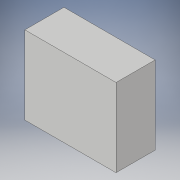
# Autodesk Inventor part: Tete
Saved by Autodesk Inventor 2019 (Build 230136000, 136)
## iProperties
Created: 2020-05-14
Part Number: Tete
Material: Générique
Document SubType Name: Modeling
Designer: qrrim
Density: 1 g/cm^3
Appearance: Par défaut
Author: qrrim
Autodesk Inventor part; units mm, degrees
ref_plane "YZ Plane" through (0, 0, 0) normal (1, 0, 0) x (0, 1, 0)
ref_plane "XZ Plane" through (0, 0, 0) normal (0, 1, 0) x (-1, 0, 0)
ref_plane "XY Plane" through (0, 0, 0) normal (0, 0, 1) x (1, 0, 0)
sketch "Esquisse1" plane through (0, 0, 0) normal (0, 0, 1) x (1, 0, 0)
  line L0 (0, 0) -> (0, 60)
  line L1 (0, 60) -> (70, 60)
  line L2 (70, 60) -> (70, 0)
  line L3 (70, 0) -> (0, 0)
  dimension "d0" = 60
  dimension "d1" = 70
  constraints: 8 end point, 3 perpendicular, 1 vertical
  measures "d0" distance of L0.start L0.end
  measures "d1" distance of L0.end L1.end
extrude "Extrusion1" add sketch "Esquisse1" along normal blind 30
shell "Coque1" thickness 1 removed faces 1 at (23.3333, 40, 0)
